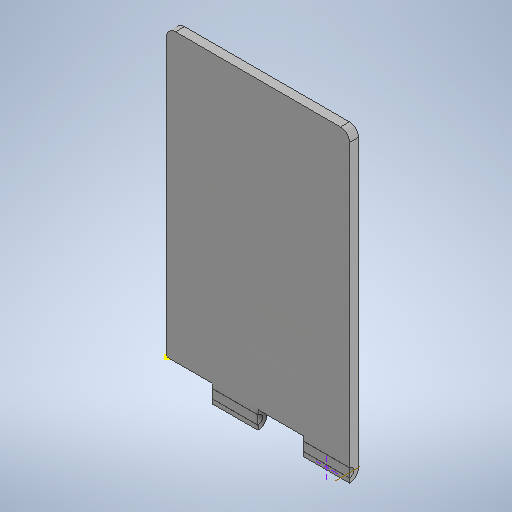
# Autodesk Inventor part: Hinge
Saved by Autodesk Inventor 2025.1 (Build 291241000, 241)
## iProperties
Created: 2024-10-22
Part Number: Hinge
Material: Generic
Document SubType Name: Modeling
Designer: vedan
Density: 1 g/cm^3
Appearance: Light Gray
Author: vedan
Autodesk Inventor part; units mm, degrees
ref_plane "YZ Plane" through (0, 0, 0) normal (1, 0, 0) x (0, 1, 0)
ref_plane "XZ Plane" through (0, 0, 0) normal (0, 1, 0) x (-1, 0, 0)
sketch "Sketch1" plane through (0, 0, 0) normal (0, 0, 1) x (1, 0, 0)
  line L0 (0, 0) -> (102.3, 0)
  line L1 (102.3, 0) -> (102.3, 160)
  line L2 (102.3, 160) -> (0, 160)
  line L3 (0, 160) -> (0, 0)
  dimension "d0" = 160
  dimension "d1" = 102.3
  constraints: 8 end point, 2 parallel, 1 horizontal, 1 perpendicular
  measures "d0" distance of L0.end L1.end
  measures "d1" distance of L1.end L2.end
extrude "Extrusion1" add sketch "Sketch1" along normal blind 5
sketch "Sketch3" plane through (102.3, 0, 0) normal (1, 0, 0) x (0, 0, -1)
  line L0 (0, 0) -> (-5, 0)
  line L1 (-5, 0) -> (-5, -5)
  line L2 (-5, -5) -> (0, -5)
  line L3 (0, -5) -> (0, 0)
  arc A0 (-5, -10) -> (-6.25, -0.1588) centre (-5, -5) ccw
  arc A1 (-5, -7.5) -> (-5, -2.5) centre (-5, -5) ccw
  line L4 (-6.25, -2.8349) -> (-6.25, -0.1588)
  line L5 (-5, 0) -> (-5, -10)
  point P0 (-5, -2.5)
  point P1 (-2.5, -5)
  dimension "d11" = 5
  dimension "d12" = 5
  dimension "d13" = 2.5
  dimension "d14" = 1.25
  constraints: 12 end point, 5 point on circle, 2 centre point, 2 parallel, 2 perpendicular, 1 coincident, 1 horizontal, 1 midpoint, 1 point on line, 1 vertical
  measures "d11" distance of L2.end L1.end
  measures "d12" distance of L1.end L0.end
  measures "d13" radial gap between concentric circles of A0 A1
  measures "d14" distance between parallel lines of L1 L4
extrude "Extrusion3" add sketch "Sketch3" against normal blind 25.575 contours L3 A0 L0 | A0 L2 A1 L1 | A0 L5 A1 L2
pattern_linear "Rectangular Pattern1" count 2 spacing 51.15 along (-1, 0, 0) of "Extrusion3"
fillet "Fillet1" radius 5 2 edges at (102.3, 160, 2.5) (0, 160, 2.5)
sketch "Sketch6" plane through (102.3, -10, 5) normal (0, 0, 1) x (1, 0, 0)
  point P0 (-102.3, 10)
  point P1 (-12.7875, 1.222)
ref_plane "Work Plane1" through (89.5125, -8.778, 5) normal (0, 0, 1) x (1, 0, 0)
sketch "Sketch7" plane through (89.5125, -8.778, 5) normal (0, 0, 1) x (1, 0, 0)
  line L0 (12.7875, 6.278) -> (-12.7875, 6.278) projected
  line L1 (12.7875, 1.278) -> (-12.7875, 1.278) projected
  line L2 (-12.7875, 6.278) -> (12.7875, 6.278)
  line L3 (12.7875, 6.278) -> (12.7875, 1.278)
  line L4 (12.7875, 1.278) -> (-12.7875, 1.278)
  line L5 (-12.7875, 1.278) -> (-12.7875, 6.278)
  point P0 (-89.5125, 8.778)
  constraints: 8 end point, 2 parallel, 1 horizontal, 1 perpendicular
extrude "Extrusion6" add sketch "Sketch7" along normal blind 0.1
pattern_linear "Rectangular Pattern2" count 2 spacing 51.2 along (-1, 0, 0) of "Extrusion6"
body "Solid1"
